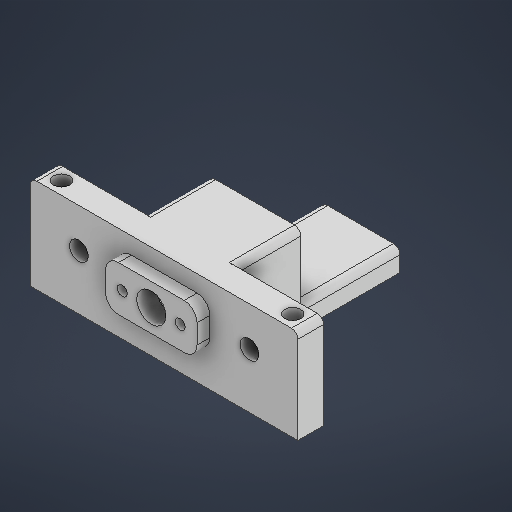
# Autodesk Inventor part: PololuMount
Saved by Autodesk Inventor 2027 (Build 310192060, 192F)
## iProperties
Created: 2026-08-09
Part Number: PololuMount
Material: Generic
Document SubType Name: Modeling
Designer: felip
Density: 1 g/cm^3
Appearance: Default
Author: felip
Autodesk Inventor part; units mm, degrees
ref_plane "YZ Plane" through (0, 0, 0) normal (1, 0, 0) x (0, 1, 0)
ref_plane "XZ Plane" through (0, 0, 0) normal (0, 1, 0) x (-1, 0, 0)
ref_plane "XY Plane" through (0, 0, 0) normal (0, 0, 1) x (1, 0, 0)
sketch "Sketch1" plane through (0, 0, 0) normal (0, 0, 1) x (1, 0, 0)
  line L0 (0, -5.1) -> (6.1, -5.1)
  line L1 (6.1, -5.1) -> (6.1, 5.1)
  line L2 (6.1, 5.1) -> (-6.1, 5.1)
  line L3 (-6.1, 5.1) -> (-6.1, -5.1)
  line L4 (-6.1, -5.1) -> (0, -5.1)
  line L5 (-6.1, 5.1) -> (-7.1, 5.1)
  line L6 (-7.1, 5.1) -> (-7.1, 6.1)
  line L7 (6.1, -5.1) -> (7.1, -5.1)
  line L8 (7.1, -5.1) -> (7.1, -6.1)
  line L9 (7.1, -6.1) -> (-7.1, -6.1)
  line L10 (-7.1, -6.1) -> (-7.1, 6.1)
  line L11 (-7.1, 6.1) -> (7.1, 6.1)
  line L12 (7.1, 6.1) -> (7.1, -6.1)
  line L13 (-7.1, -6.1) -> (7.1, -6.1)
  line L14 (7.1, -6.1) -> (7.1, -9.5)
  line L15 (7.1, -9.5) -> (-7.1, -9.5)
  line L16 (-7.1, -9.5) -> (-7.1, -6.1)
  line L17 (-6.1, -5.1) -> (-6.1, -9.5)
  line L18 (6.1, -5.1) -> (6.1, -9.5)
  point P0 (0, 0)
  point P1 (6.1, -6.1)
  point P2 (-6.1, -6.1)
  dimension "d0" = 5.1
  dimension "d1" = 6.1
  dimension "d2" = 10.2
  dimension "d3" = 12.2
  dimension "d4" = 10.2
  dimension "d5" = 1
  dimension "d6" = 1
  dimension "d7" = 1
  dimension "d8" = 1
  dimension "d9" = 3.4
  constraints: 38 end point, 9 perpendicular, 4 horizontal, 4 parallel, 2 point on line
  measures "d0" distance of point (0, 0) L0.start
  measures "d1" distance of L0.start L0.end
  measures "d2" distance of L0.end L1.end
  measures "d3" distance of L1.end L2.end
  measures "d4" distance of L2.end L3.end
  measures "d5" distance of L2.end L5.end
  measures "d6" distance of L5.end L6.end
  measures "d7" distance of L0.end L7.end
  measures "d8" distance of L7.end L8.end
  measures "d9" distance of L13.end L14.end
extrude "Extrusion1" add sketch "Sketch1" against normal blind 32.5 contours L18 L15 L17 L9
extrude "Extrusion2" add sketch "Sketch1" against normal blind 13.1 contours L0 L18 L9 L17 L4 | L1 L2 L5 L6 L11 L12 L7 | L7 L8 L9 L18 | L17 L9 L10 L5 L3 | L9 L14 L15 L18 | L17 L15 L16 L9
sketch "Sketch2" plane through (0, 0, 0) normal (0, 0, 1) x (1, 0, 0)
  line L0 (-7.1, -9.5) -> (-7.1, 6.1) projected
  line L1 (7.1, 6.1) -> (7.1, -9.5) projected
  line L2 (-7.1, 6.1) -> (7.1, 6.1)
  line L3 (7.1, 6.1) -> (7.1, -9.5)
  line L4 (7.1, -9.5) -> (-7.1, -9.5)
  line L5 (-7.1, -9.5) -> (-7.1, 6.1)
  point P0 (0, 0)
  constraints: 8 end point, 2 parallel, 1 horizontal, 1 perpendicular
extrude "Extrusion3" add sketch "Sketch2" against normal blind 1
sketch "Sketch3" plane through (0, 0, 0) normal (0, 0, 1) x (-1, 0, 0)
  line L0 (-6.1, 5.1) -> (-6.1, -5.1) projected
  line L1 (-6.1, 5.1) -> (6.1, -5.1)
  line L2 (6.1, 5.1) -> (-6.1, 5.1) projected
  line L3 (6.1, 5.1) -> (-6.1, 5.1) projected
  line L4 (6.1, 5.1) -> (-6.1, -5.1)
  circle A0 centre (0, 0) radius 2.25
  line L5 (0, 0) -> (4.5, 0)
  line L6 (7.1, 6.1) -> (7.1, -9.5) projected
  line L7 (0, 0) -> (-4.5, 0)
  circle A1 centre (-4.5, 0) radius 0.775
  circle A2 centre (4.5, 0) radius 0.775
  dimension "d19" = 4.5
  dimension "d20" = 4.5
  dimension "d21" = 4.5
  dimension "d22" = 1.55
  dimension "d23" = 1.55
  constraints: 8 end point, 3 centre point, 3 coincident, 2 midpoint, 1 horizontal, 1 perpendicular, 1 other
  measures "d19" diameter of A0
  measures "d20" distance of L5.start L5.end
  measures "d21" distance of L7.start L7.end
  measures "d22" diameter of A1
  measures "d23" diameter of A2
extrude "Extrusion4" cut sketch "Sketch3" against normal blind 6 contours A0 L4 L1 | L1 L7 A0 | A0 L7 L4 | L4 L1 A0 | L5 A0 L1 | L4 A0 L5 | A1 | A2
sketch "Sketch4" plane through (0, 0, -1) normal (0, 0, -1) x (1, 0, 0)
  line L0 (0, 0) -> (0, 3.5)
  line L1 (0, 0) -> (0, -3.5)
  line L2 (0, -3.5) -> (7.1, -3.5)
  line L3 (-7.1, 6.1) -> (-7.1, -9.5) projected
  line L4 (7.1, -3.5) -> (-7.1, -3.5)
  line L5 (-7.1, -3.5) -> (-7.1, 3.5)
  line L6 (-7.1, 3.5) -> (7.1, 3.5)
  line L7 (7.1, 3.5) -> (7.1, -3.5)
  circle A0 centre (0, 0) radius 2.25
  line L8 (0, 0) -> (-4.5, 0)
  circle A1 centre (4.5, 0) radius 0.775 projected
  line L9 (0, 0) -> (4.5, 0)
  circle A2 centre (4.5, 0) radius 0.775
  circle A3 centre (-4.5, 0) radius 0.8
  dimension "d26" = 3.5
  dimension "d27" = 3.5
  dimension "d28" = 7.1
  dimension "d29" = 4.5
  dimension "d30" = 4.5
  constraints: 18 end point, 3 centre point, 3 coincident, 3 horizontal, 2 parallel, 2 perpendicular, 2 vertical, 1 concentric, 1 point on line
  measures "d26" distance of L0.start L0.end
  measures "d27" distance of L0.start L1.end
  measures "d28" distance of L1.end L2.end
  measures "d29" diameter of A0
  measures "d30" distance of L8.start L8.end
extrude "Extrusion5" add sketch "Sketch4" against normal blind 3 contours A0 L1 L4 L3 L6 L0 | L0 L6 L7 L2 L1 A0
sketch "Sketch5" plane through (-7.1, -9.5, -13.1) normal (-1, 0, 0) x (0, 0, 1)
  line L0 (13.1, 15.6) -> (0, 15.6) projected
  line L1 (13.6, 15.6) -> (13.1, 15.6)
  line L2 (0, 0) -> (13.6, 0) projected
  line L3 (13.1, 15.6) -> (9.1, 15.6)
  line L4 (9.1, 15.6) -> (9.1, 0)
  line L5 (9.1, 0) -> (13.1, 0)
  line L6 (13.1, 0) -> (13.1, 15.6)
  point P0 (13.1, 9.5)
  dimension "d33" = 0.5
  dimension "d34" = 4
  constraints: 11 end point, 2 parallel, 1 horizontal, 1 perpendicular, 1 point on line
  measures "d33" distance of L1.start L0.start
  measures "d34" distance of L5.end L4.end
extrude "Extrusion6" add sketch "Sketch5" along normal blind 13.65
sketch "Sketch7" plane through (7.1, -9.5, -13.1) normal (1, 0, 0) x (0, 0, -1)
  line L0 (-13.1, 15.6) -> (0, 15.6) projected
  line L1 (-13.1, 0) -> (0, 0) projected
  line L2 (-13.1, 15.6) -> (-9.1, 15.6)
  line L3 (-9.1, 15.6) -> (-9.1, 0)
  line L4 (-9.1, 0) -> (-13.1, 0)
  line L5 (-13.1, 0) -> (-13.1, 15.6)
  point P0 (-13.1, 9.5)
  dimension "d42" = 4
  constraints: 8 end point, 2 parallel, 1 horizontal, 1 perpendicular, 1 point on line
  measures "d42" distance of L3.end L4.end
extrude "Extrusion7" add sketch "Sketch7" along normal blind 13.65
sketch "Sketch8" plane through (0, 0, 2) normal (0, 0, 1) x (1, 0, 0)
  circle A0 centre (0, 0) radius 2.25 projected
  line L0 (0, 0) -> (13.25, 0)
  line L1 (0, 0) -> (-13.25, 0)
  circle A1 centre (-13.25, 0) radius 1.45
  circle A2 centre (13.25, 0) radius 1.45
  dimension "d45" = 13.25
  dimension "d46" = 13.25
  dimension "d47" = 2.9
  dimension "d48" = 2.9
  constraints: 4 end point, 2 centre point, 2 coincident, 2 horizontal
  measures "d45" distance of L0.start L0.end
  measures "d46" distance of L0.start L1.end
  measures "d47" diameter of A1
  measures "d48" diameter of A2
extrude "Extrusion8" cut sketch "Sketch8" against normal blind 13.65 contours A1 | A2
sketch "Sketch11" plane through (-7.1, 6.1, -13.1) normal (0, 1, 0) x (1, 0, 0)
  line L0 (0, -9.1) -> (-13.65, -9.1) projected
  line L1 (0, -9.1) -> (-7.6, -9.1)
  line L2 (-7.6, -9.1) -> (-7.6, -11.1)
  line L3 (-7.6, -13.1) -> (-7.6, -9.1) projected
  line L4 (-7.6, -11.1) -> (-9.6, -11.1)
  line L5 (-9.6, -11.1) -> (-10.6, -11.1)
  line L6 (-10.6, -11.1) -> (-10.85, -11.1)
  circle A0 centre (-10.85, -11.1) radius 1.25
  line L7 (14.2, -9.1) -> (14.2, 0) projected
  line L8 (14.2, -9.1) -> (21.8, -9.1)
  line L9 (14.2, -9.1) -> (27.85, -9.1) projected
  line L10 (21.8, -9.1) -> (25.05, -9.1)
  line L11 (14.2, -9.1) -> (27.85, -9.1) projected
  line L12 (25.05, -9.1) -> (25.05, -11.1)
  circle A1 centre (25.05, -11.1) radius 1.25
  point P0 (7.1, -13.1)
  dimension "d52" = 7.6
  dimension "d53" = 2
  dimension "d54" = 2
  dimension "d55" = 1
  dimension "d56" = 0.25
  dimension "d57" = 7.6
  dimension "d58" = 3.25
  dimension "d59" = 2
  dimension "d60" = 2.5
  constraints: 16 end point, 4 point on line, 2 coincident, 2 horizontal, 1 centre point, 1 horizontal alignment, 1 midpoint, 1 perpendicular, 2 other
  measures "d52" distance of L0.start L1.end
  measures "d53" distance of L1.end L2.end
  measures "d54" distance of L2.end L4.end
  measures "d55" distance of L4.end L5.end
  measures "d56" distance of L5.end L6.end
  measures "d57" distance of L7.start L8.end
  measures "d58" distance of L8.end L10.end
  measures "d59" distance of L10.end L12.end
  measures "d60" diameter of A1
extrude "Extrusion9" cut sketch "Sketch11" against normal blind 20
sketch "Sketch12" plane through (20.75, -9.5, -13.1) normal (1, 0, 0) x (0, 0, -1)
  line L0 (-9.1, 0) -> (-13.1, 0) projected
  line L1 (19.4, 0) -> (19.4, 3.4) projected
  line L2 (-13.1, 0) -> (19.4, 0)
  line L3 (19.4, 0) -> (19.4, 1)
  line L4 (19.4, 1) -> (-13.1, 1)
  line L5 (-13.1, 1) -> (-13.1, 0)
  point P0 (-13.1, 9.5)
  dimension "d63" = 1
  constraints: 8 end point, 2 parallel, 1 horizontal, 1 perpendicular, 1 point on line
  measures "d63" distance of L3.end L2.end
extrude "Extrusion10" cut sketch "Sketch12" against normal blind 50
sketch "Sketch13" plane through (0, 0, -13.1) normal (0, 0, -1) x (-1, 0, 0)
  line L0 (6.1, -5.1) -> (-6.1, -5.1) projected
  line L1 (6.1, -8.5) -> (6.1, -6.1) projected
  line L2 (-6.1, -5.1) -> (6.1, -5.1)
  line L3 (6.1, -5.1) -> (6.1, -6.1)
  line L4 (6.1, -6.1) -> (-6.1, -6.1)
  line L5 (-6.1, -6.1) -> (-6.1, -5.1)
  point P0 (0, 0)
  constraints: 8 end point, 2 parallel, 1 horizontal, 1 perpendicular
extrude "Extrusion11" add sketch "Sketch13" along normal blind 19.4
sketch "Sketch14" plane through (0, 0, -13.1) normal (0, 0, -1) x (-1, 0, 0)
  line L0 (-7.1, 6.1) -> (-7.1, -8.5) projected
  line L1 (20.75, -8.5) -> (-20.75, -8.5) projected
  line L2 (-7.1, 6.1) -> (-6.1, 6.1)
  line L3 (-6.1, 6.1) -> (-6.1, -8.5)
  line L4 (-6.1, -8.5) -> (-7.1, -8.5)
  line L5 (-7.1, -8.5) -> (-7.1, 6.1)
  line L6 (7.1, -8.5) -> (7.1, 6.1) projected
  line L7 (-7.1, 6.1) -> (7.1, 6.1)
  line L8 (7.1, 6.1) -> (7.1, 5.1)
  line L9 (7.1, 5.1) -> (-7.1, 5.1)
  line L10 (-7.1, 5.1) -> (-7.1, 6.1)
  line L11 (7.1, 6.1) -> (6.1, 6.1)
  line L12 (6.1, 6.1) -> (6.1, -8.5)
  line L13 (6.1, -8.5) -> (7.1, -8.5)
  line L14 (7.1, -8.5) -> (7.1, 6.1)
  point P0 (0, 0)
  point P1 (-6.1, 5.1)
  point P2 (6.1, 5.1)
  dimension "d68" = 1
  dimension "d69" = 1
  dimension "d70" = 1
  constraints: 24 end point, 6 parallel, 3 horizontal, 3 perpendicular, 3 point on line
  measures "d68" distance of L3.end L4.end
  measures "d69" distance of L7.end L8.end
  measures "d70" distance of L13.end L12.end
extrude "Extrusion12" add sketch "Sketch14" along normal blind 1 contours L2 L3 L9 L0 | L9 L3 L1 L0 | L7 L12 L9 L3 | L7 L6 L9 L12 | L9 L6 L1 L12
fillet "Fillet4" radius 2 4 edges at (-7.1, 3.5, 1) (7.1, 3.5, 1) (7.1, -3.5, 1) (-7.1, -3.5, 1)
fillet "Fillet5" radius 1 2 edges at (-7.1, 6.1, -9.05) (7.1, 6.1, -9.05)
fillet "Fillet6" radius 0.5 2 edges at (-6.1, 5.1, -7.55) (6.1, 5.1, -7.55)
fillet "Fillet7" radius 1 2 edges at (-20.75, 6.1, -2) (20.75, 6.1, -2)
fillet "Face Fillet1" radius 1 1 edges at (6.1, -6.8, -14.1)
fillet "Face Fillet2" radius 1 1 edges at (-6.1, -6.8, -14.1)
fillet "Fillet8" radius 1 3 edges at (6.1, -5.1, -23.8) (6.3929, -5.1, -14.3929) (6.5999, -5.1, -14.1)
fillet "Fillet9" radius 1 3 edges at (-6.1, -5.1, -23.8) (-6.3929, -5.1, -14.3929) (-6.5999, -5.1, -14.1)
sketch "Sketch16" plane through (0, 0, 2) normal (0, 0, 1) x (1, 0, 0)
  circle A0 centre (-4.5, 0) radius 0.775 projected
  circle A1 centre (-4.5, 0) radius 0.775
  circle A2 centre (-4.5, 0) radius 0.8
  point P0 (0, 0)
  constraints: 2 centre point, 2 coincident
extrude "Extrusion14" add sketch "Sketch16" against normal blind 3
sketch "Sketch17" plane through (6.1, -8.5, -15.1) normal (1, 0, 0) x (0, 0, -1)
  line L0 (17.4, 2.4) -> (17.4, 0) projected
  line L1 (17.4, 3.4) -> (0, 3.4) projected
  line L2 (17.4, 0) -> (15.4, 0)
  line L3 (15.4, 0) -> (15.4, 3.4)
  line L4 (15.4, 3.4) -> (17.4, 3.4)
  line L5 (17.4, 3.4) -> (17.4, 0)
  point P0 (-15.1, 8.5)
  dimension "d86" = 2
  constraints: 8 end point, 2 parallel, 1 horizontal, 1 perpendicular, 1 point on line
  measures "d86" distance of L3.end L4.end
extrude "Extrusion15" cut sketch "Sketch17" against normal blind 13
body "Solid1"
